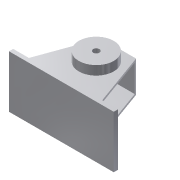
# Autodesk Inventor part: Casing
Saved by Autodesk Inventor 2016 (Build 200138000, 138)
## iProperties
Created: 2015-05-18
Part Number: Casing
Material: Generic
Document SubType Name: Modeling
Designer: Andy
Density: 1 g/cm^3
Appearance: Default
Author: Andy
Autodesk Inventor part; units mm, degrees
ref_plane "YZ Plane" through (0, 0, 0) normal (1, 0, 0) x (0, 1, 0)
ref_plane "XZ Plane" through (0, 0, 0) normal (0, 1, 0) x (-1, 0, 0)
ref_plane "XY Plane" through (0, 0, 0) normal (0, 0, 1) x (1, 0, 0)
sketch "Sketch1" plane through (0, 0, 0) normal (0, 1, 0) x (-1, 0, 0)
  line L0 (0, 0) -> (150, 0)
  line L1 (150, 0) -> (150, -75)
  line L2 (150, -75) -> (0, -75)
  line L3 (0, -75) -> (0, 0)
  dimension "d0" = 150
  dimension "d1" = 75
  constraints: 8 end point, 2 parallel, 1 horizontal, 1 perpendicular
  measures "d0" distance of L0.start L0.end
  measures "d1" distance of L0.end L1.end
extrude "Extrusion1" add sketch "Sketch1" along normal blind 6
sketch "Sketch6" plane through (-150, 0, 0) normal (0, 0, 1) x (1, 0, 0)
  line L0 (0, 6) -> (150, 6) projected
  line L1 (50, 82) -> (22.5, 6)
  line L2 (100, 82) -> (127.5, 6)
  line L3 (50, 82) -> (100, 82)
  line L4 (22.5, 6) -> (127.5, 6)
  line L5 (22.5, 6) -> (127.5, 6)
  line L6 (100, 82) -> (50, 82)
  line L7 (50, 82) -> (22.5, 6)
  line L8 (100, 82) -> (127.5, 6)
  constraints: 16 end point, 4 collinear, 1 parallel
extrude "Extrusion2" add sketch "Sketch6" against normal blind 45
sketch "Sketch7" plane through (-150, 0, 0) normal (0, 0, 1) x (1, 0, 0)
  line L0 (150, 0) -> (0, 0) projected
  line L1 (75, 0) -> (75, 50)
  circle A0 centre (75, 50) radius 25
  dimension "d14" = 50
  dimension "d15" = 50
  constraints: 2 end point, 1 centre point, 1 coincident, 1 midpoint, 1 vertical
  measures "d14" distance of L1.start L1.end
  measures "d15" diameter of A0
extrude "Extrusion3" add sketch "Sketch7" along normal blind 13
sketch "Sketch9" plane through (0, 0, 0) normal (1, 0, 0) x (0, 0, -1)
  line L0 (0, 6) -> (75, 6) projected
  line L1 (45, 82) -> (0, 82)
  line L2 (0, 82) -> (45, 82) projected
  line L3 (0, 6) -> (0, 9)
  line L4 (0, 6) -> (0, 82) projected
  line L5 (0, 9) -> (45, 9)
  line L6 (45, 6) -> (45, 82) projected
  line L7 (0, 82) -> (3, 82)
  line L8 (3, 82) -> (3, 9)
  line L9 (0, 82) -> (0, 79)
  line L10 (0, 79) -> (45, 79)
  line L11 (45, 79) -> (42, 79)
  line L12 (42, 79) -> (42, 6)
  line L13 (3, 9) -> (3, 79)
  line L14 (3, 79) -> (42, 79)
  line L15 (42, 79) -> (42, 9)
  line L16 (42, 9) -> (3, 9)
  dimension "d18" = 3
  dimension "d19" = 3
  dimension "d20" = 3
  dimension "d21" = 3
  constraints: 26 end point, 10 point on line, 5 perpendicular, 3 equal length
  measures "d18" distance of L0.start L3.end
  measures "d19" distance of L1.end L7.end
  measures "d20" distance of L1.end L9.end
  measures "d21" distance of L10.end L11.end
extrude "Extrusion4" cut sketch "Sketch9" against normal blind 150 contours L5 L8 L10 L12
sketch "Sketch10" plane through (-75, 50, 13) normal (0, 0, 1) x (1, 0, 0)
  circle A0 centre (0, 0) radius 25 projected
  circle A1 centre (0, 0) radius 4.5
  point P0 (75, -50)
  dimension "d24" = 9
  constraints: 1 centre point, 1 coincident
  measures "d24" diameter of A1
extrude "Extrusion5" cut sketch "Sketch10" against normal blind 150 contours A1
body "Solid1"
